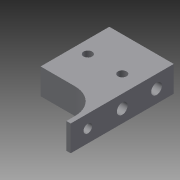
# Autodesk Inventor part: 34Assembly
Saved by Autodesk Inventor 2015 (Build 190159000, 159)
## iProperties
Created: 2015-02-01
Part Number: 34Assembly
Material: Generic
Document SubType Name: Modeling
Designer: whitaus15
Density: 1 g/cm^3
Appearance: Default
Author: whitaus15
Autodesk Inventor part; units mm, degrees
ref_plane "YZ Plane" through (0, 0, 0) normal (1, 0, 0) x (0, 1, 0)
ref_plane "XZ Plane" through (0, 0, 0) normal (0, 1, 0) x (-1, 0, 0)
ref_plane "XY Plane" through (0, 0, 0) normal (0, 0, 1) x (1, 0, 0)
sketch "Sketch1" plane through (0, 0, 0) normal (0, 1, 0) x (-1, 0, 0)
  line L0 (0, 0) -> (47.625, 0)
  line L1 (47.625, 0) -> (47.625, -76.2)
  line L2 (47.625, -76.2) -> (0, -76.2)
  line L3 (0, -76.2) -> (0, 0)
  dimension "d0" = 47.625
  dimension "d1" = 76.2
  constraints: 8 end point, 2 parallel, 1 horizontal, 1 perpendicular
  measures "d0" distance of L0.start L0.end
  measures "d1" distance of L0.end L1.end
extrude "Extrusion1" add sketch "Sketch1" along normal blind 19.05
sketch "Sketch2" plane through (-47.625, 0, -76.2) normal (-1, 0, 0) x (0, 0, 1)
  line L0 (0, 0) -> (0, 19.05) projected
  line L1 (0, 19.05) -> (76.2, 19.05) projected
  line L2 (76.2, 0) -> (0, 0) projected
  line L3 (48.9575, 0) -> (51.7141, 0) projected
  line L4 (51.7141, 0) -> (51.7141, 9.525) projected
  line L5 (51.7141, 9.525) -> (48.9575, 9.525) projected
  line L6 (48.9575, 9.525) -> (48.9575, 0) projected
  line L7 (0, 0) -> (76.2, 0) projected
  line L8 (0, 9.525) -> (50.8, 9.525)
  line L9 (0, 9.525) -> (25.4, 9.525)
  line L10 (76.2, 0) -> (76.2, 19.05) projected
  line L11 (50.8, 9.525) -> (38.1, 9.525)
  line L12 (25.4, 9.525) -> (12.7, 9.525)
  circle A0 centre (38.1, 9.525) radius 3.9688
  circle A1 centre (12.7, 9.525) radius 3.9688
  point P0 (53.975, 9.525)
  point P1 (53.975, 0)
  dimension "d8" = 50.8
  dimension "d9" = 25.4
  dimension "d10" = 7.9375
  dimension "d11" = 7.9375
  constraints: 8 end point, 3 midpoint, 2 centre point, 2 coincident, 1 horizontal, 1 point on line, 1 other
  measures "d8" distance of L8.start L8.end
  measures "d9" distance of L8.start L9.end
  measures "d10" diameter of A0
  measures "d11" diameter of A1
sketch "Sketch3" plane through (-47.625, 0, -76.2) normal (-1, 0, 0) x (0, 0, 1)
  line L0 (76.2, 19.05) -> (50.8, 19.05)
  line L1 (50.8, 19.05) -> (50.8, 0)
  line L2 (50.8, 0) -> (76.2, 0)
  line L3 (76.2, 0) -> (76.2, 19.05)
  point P0 (76.2, 0)
  dimension "d21" = 25.4
  dimension "d27" = 19.05
  constraints: 8 end point, 2 parallel, 1 horizontal, 1 perpendicular
  measures "d21" distance of L0.start L0.end
  measures "d27" distance of L0.end L1.end
extrude "Extrusion3" cut sketch "Sketch3" against normal blind 44.45
fillet "Fillet4" radius 19.05 1 edges at (-3.175, 9.525, -25.4)
extrude "Extrusion4" cut sketch "Sketch2" against normal through all contours A1 L8 | L8 A1 | A0 L8 | L8 A0
sketch "Sketch5" plane through (-3.175, 0, -76.2) normal (-1, 0, 0) x (0, 0, 1)
  line L0 (50.8, 0) -> (50.8, 19.05) projected
  line L1 (76.2, 19.05) -> (76.2, 0) projected
  line L2 (76.2, 9.525) -> (63.5, 9.525)
  circle A0 centre (63.5, 9.525) radius 3.175
  dimension "d28" = 12.7
  dimension "d29" = 6.35
  constraints: 2 end point, 1 centre point, 1 coincident, 1 horizontal, 1 midpoint
  measures "d28" distance of L2.start L2.end
  measures "d29" diameter of A0
extrude "Extrusion5" cut sketch "Sketch5" along normal mid plane 44.45
sketch "Sketch6" plane through (-3.175, 0, -76.2) normal (-1, 0, 0) x (0, 0, 1)
  spline S0 degree 2 poles (66.675, 9.525) (66.675, 15.0243) (61.9125, 12.2746) (57.15, 9.525) (61.9125, 6.7754) (66.675, 4.0257) (66.675, 9.525) knots 0 0 0 0.333333 0.333333 0.666667 0.666667 1 1 1 weights 1 0.5 1 0.5 1 0.5 1 projected
  line L0 (76.2, 0) -> (76.2, 19.05) projected
  line L1 (76.2, 9.525) -> (63.5, 9.525)
  circle A0 centre (63.5, 9.525) radius 4.7625
  dimension "d33" = 12.7
  dimension "d34" = 9.525
  constraints: 2 end point, 1 centre point, 1 coincident, 1 horizontal, 1 midpoint, 1 other
  measures "d33" distance of L1.start L1.end
  measures "d34" diameter of A0
extrude "Extrusion6" cut sketch "Sketch6" along normal through all
sketch "Sketch7" plane through (0, 19.05, 0) normal (0, 1, 0) x (1, 0, 0)
  line L0 (-47.625, 25.4) -> (-47.625, 50.8)
  line L1 (-47.625, 50.8) -> (-38.1, 50.8)
  circle A0 centre (-38.1, 50.8) radius 3.175
  line L2 (-38.1, 50.8) -> (-12.7, 50.8)
  circle A1 centre (-12.7, 50.8) radius 3.175
  point P0 (0, 0)
  dimension "d37" = 25.4
  dimension "d38" = 9.525
  dimension "d39" = 6.35
  dimension "d40" = 25.4
  dimension "d41" = 6.35
  constraints: 6 end point, 2 centre point, 2 coincident, 1 horizontal, 1 perpendicular, 1 vertical
  measures "d37" distance of L0.start L0.end
  measures "d38" distance of L0.end L1.end
  measures "d39" diameter of A0
  measures "d40" distance of L2.start L2.end
  measures "d41" diameter of A1
extrude "Extrusion7" cut sketch "Sketch7" against normal blind 25.4
body "Solid1"
